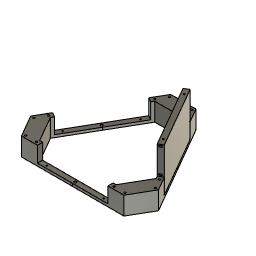
mpminideltaBase v6 (Autodesk Fusion 360 design; units mm, degrees)
Autodesk Fusion 360 part; units mm, degrees
sketch "Sketch1" plane through (0, 0, 0) normal (0, 0, 1) x (1, 0, 0)
  line L0 (0, 128.5246) -> (24.5, 128.5246)
  line L1 (24.5, 128.5246) -> (33.9962, 112.0679)
  line L2 (33.9962, 112.0679) -> (22.7364, 105.5705)
  line L3 (22.7364, 105.5705) -> (0, 105.5705)
  circle A0 centre (0, 0) radius 15
  line L4 (24.5, 128.5246) -> (25.9994, 125.9262)
  line L5 (24.5, 128.5246) -> (21.5, 128.5246)
  line L6 (33.9962, 112.0679) -> (29.6655, 109.5689)
  line L7 (33.9962, 112.0679) -> (36.4952, 107.7372)
  circle A1 centre (21.5, 123.3299) radius 1.75
  circle A2 centre (32.1825, 105.2486) radius 1.75
  line L8 (36.4952, 107.7372) -> (44.2521, 94.2946)
  line L9 (36.4952, 107.7372) -> (45.6165, 91.9302)
  line L10 (47.3658, 88.8987) -> (43.0351, 86.3997)
  line L11 (41.2858, 89.4312) -> (45.6165, 91.9302)
  arc A3 (41.2858, 89.4312) -> (43.0351, 86.3997) centre (42.1605, 87.9154) ccw
  line L12 (36.4952, 107.7372) -> (45.6165, 91.9302)
  line L13 (47.3658, 88.8987) -> (48.5676, 86.8161)
  line L14 (24.5, 128.5246) -> (45.6165, 91.9302)
  line L15 (47.3658, 88.8987) -> (74, 42.7422)
  line L16 (36.4952, 107.7372) -> (45.6165, 91.9302)
  line L17 (47.3658, 88.8987) -> (48.5676, 86.8161)
  line L18 (21.5, 123.3299) -> (21.4713, 123.3133)
  line L19 (-47.3658, 88.8987) -> (-74, 42.7422)
  line L20 (-47.3658, 88.8987) -> (-43.0351, 86.3997)
  arc A4 (-43.0351, 86.3997) -> (-41.2858, 89.4312) centre (-42.1605, 87.9154) ccw
  line L21 (-41.2858, 89.4312) -> (-45.6165, 91.9302)
  line L22 (-36.4952, 107.7372) -> (-45.6165, 91.9302)
  line L23 (-24.5, 128.5246) -> (-45.6165, 91.9302)
  circle A5 centre (-32.1825, 105.2486) radius 1.75
  line L24 (-33.9962, 112.0679) -> (-22.7364, 105.5705)
  line L25 (-22.7364, 105.5705) -> (0, 105.5705)
  circle A6 centre (-21.5, 123.3299) radius 1.75
  line L26 (0, 128.5246) -> (-24.5, 128.5246)
  line L27 (-53.3056, -85.4693) -> (-0.0159, -85.457)
  arc A7 (-53.3067, -80.4693) -> (-56.8067, -80.4701) centre (-55.0567, -80.4697) ccw
  line L28 (-56.8067, -80.4701) -> (-56.8056, -85.4701)
  line L29 (-53.3056, -85.4693) -> (-53.3067, -80.4693)
  line L30 (-98.0926, -8.961) -> (-102.4221, -6.46)
  line L31 (-100.6714, -3.4293) -> (-99.4687, -1.3473)
  arc A8 (-98.0926, -8.961) -> (-96.3419, -5.9303) centre (-97.2172, -7.4457) ccw
  line L32 (-100.6714, -3.4293) -> (-96.3419, -5.9303)
  line L33 (-100.6714, -3.4293) -> (-99.4687, -1.3473)
  line L34 (-100.6714, -3.4293) -> (-74.0159, 42.7148)
  line L35 (-111.5508, -22.2629) -> (-103.7876, -8.8238)
  circle A9 centre (-107.2392, -24.7535) radius 1.75
  line L36 (-114.0518, -26.5924) -> (-111.5508, -22.2629)
  line L37 (-123.5556, -43.0447) -> (-114.0518, -26.5924)
  circle A10 centre (-117.5568, -43.0454) radius 1.75
  line L38 (-111.3056, -64.2623) -> (-123.5556, -43.0447)
  line L39 (-111.3056, -64.2623) -> (-99.0556, -85.4799)
  line L40 (-99.0556, -85.4799) -> (-56.8056, -85.4701)
  circle A11 centre (-96.0568, -80.2845) radius 1.75
  circle A12 centre (-75.0567, -80.4951) radius 1.75
  line L41 (-80.0556, -85.4755) -> (-80.0586, -72.4755)
  line L42 (-80.0586, -72.4755) -> (-91.4268, -52.7853)
  line L43 (-102.7949, -33.095) -> (-91.4268, -52.7853)
  line L44 (-114.0518, -26.5924) -> (-102.7949, -33.095)
  line L45 (100.6714, -3.4293) -> (74.0159, 42.7148)
  arc A13 (96.3419, -5.9303) -> (98.0926, -8.961) centre (97.2172, -7.4457) ccw
  line L46 (98.0926, -8.961) -> (102.4221, -6.46)
  line L47 (100.6714, -3.4293) -> (96.3419, -5.9303)
  line L48 (56.8067, -80.4701) -> (56.8056, -85.4701)
  line L49 (53.3056, -85.4693) -> (50.9011, -85.4688)
  arc A14 (56.8067, -80.4701) -> (53.3067, -80.4693) centre (55.0567, -80.4697) ccw
  line L50 (53.3056, -85.4693) -> (53.3067, -80.4693)
  line L51 (53.3056, -85.4693) -> (50.9011, -85.4688)
  line L52 (53.3056, -85.4693) -> (0.0159, -85.457)
  line L53 (75.0556, -85.4744) -> (59.5355, -85.4708)
  circle A15 centre (75.0567, -80.4951) radius 1.75
  line L54 (80.0556, -85.4755) -> (75.0556, -85.4744)
  line L55 (99.0556, -85.4799) -> (80.0556, -85.4755)
  circle A16 centre (96.0568, -80.2845) radius 1.75
  line L56 (111.3056, -64.2623) -> (99.0556, -85.4799)
  line L57 (111.3056, -64.2623) -> (123.5556, -43.0447)
  line L58 (123.5556, -43.0447) -> (102.4221, -6.46)
  circle A17 centre (117.5568, -43.0454) radius 1.75
  circle A18 centre (107.2392, -24.7535) radius 1.75
  line L59 (114.0518, -26.5924) -> (102.7949, -33.095)
  line L60 (102.7949, -33.095) -> (91.4268, -52.7853)
  line L61 (80.0586, -72.4755) -> (91.4268, -52.7853)
  line L62 (80.0556, -85.4755) -> (80.0586, -72.4755)
  line L63 (-103.7876, -8.8238) -> (-102.4221, -6.46)
  line L64 (56.8056, -85.4701) -> (59.5355, -85.4708)
  circle A19 centre (-69.6693, 40.2432) radius 2.25
  circle A20 centre (-0.017, -80.457) radius 2.25
  circle A21 centre (69.6863, 40.2138) radius 2.25
  line L65 (-102.4221, -6.46) -> (-100.6714, -3.4293)
  line L66 (-47.3658, 88.8987) -> (-45.6165, 91.9302)
  line L67 (45.6165, 91.9302) -> (47.3658, 88.8987)
  line L68 (100.6714, -3.4293) -> (102.4221, -6.46)
  line L69 (53.3056, -85.4693) -> (56.8056, -85.4701)
  line L70 (-56.8056, -85.4701) -> (-53.3056, -85.4693)
  line L71 (-38.7044, 83.9007) -> (-65.3386, 37.7442)
  line L72 (-38.7044, 83.9007) -> (-36.9551, 86.9322)
  line L73 (-18.725, 118.5246) -> (-36.9551, 86.9322)
  line L74 (0, 118.5246) -> (-18.725, 118.5246)
  line L75 (0, 118.5246) -> (18.725, 118.5246)
  line L76 (18.725, 118.5246) -> (25.3348, 107.0699)
  line L77 (25.3348, 107.0699) -> (27.8338, 102.7392)
  line L78 (27.8338, 102.7392) -> (36.9551, 86.9322)
  line L79 (36.9551, 86.9322) -> (38.7044, 83.9007)
  line L80 (38.7044, 83.9007) -> (60.3427, 46.402)
  line L81 (60.3427, 46.402) -> (111.9829, -43.0892)
  line L82 (102.6453, -59.2623) -> (112.0078, -43.046)
  line L83 (53.3079, -75.4693) -> (10.014, -75.4593)
  line L84 (53.3079, -75.4693) -> (93.2882, -75.4693)
  line L85 (102.6453, -59.2623) -> (93.2882, -75.4693)
  line L86 (-102.6453, -59.2623) -> (-112.0078, -43.046)
  line L87 (-112.0078, -43.046) -> (-105.3927, -31.5944)
  line L88 (-102.6453, -59.2623) -> (-93.2802, -75.4832)
  line L89 (-105.3927, -31.5944) -> (-65.3386, 37.7442)
  line L90 (10.014, -75.4593) -> (-93.2802, -75.4832)
  line L91 (-12.9851, 7.5092) -> (12.9946, -7.4927)
  line L92 (-0.0084, 15) -> (-0.0106, -15)
  line L93 (12.9957, 7.4908) -> (-12.9862, -7.5073)
  circle A22 centre (-106.9755, -61.7623) radius 2.25
  circle A23 centre (106.9755, -61.7623) radius 2.25
  line L94 (0, 128.5246) -> (0, 118.5246)
  circle A24 centre (0, 123.5246) radius 2.25
  line L95 (-33.9962, 112.0679) -> (-29.6655, 109.5689)
  line L96 (0, 123.5246) -> (21.6125, 123.5246)
  line L97 (-21.6125, 123.5246) -> (-29.6655, 109.5689)
  line L98 (-5, 123.5246) -> (-21.6125, 123.5246)
  line L99 (-5, 123.5246) -> (-2.25, 123.5246)
  line L100 (-19.7609, 123.5246) -> (-13.7609, 123.5246)
  line L101 (-22.5379, 121.9209) -> (-25.5367, 116.724)
  circle A25 centre (-25.5367, 116.724) radius 2.25
  circle A26 centre (-13.7609, 123.5246) radius 2.25
  line L102 (21.6125, 123.5246) -> (41.2858, 89.4312)
  line L103 (22.5379, 121.9209) -> (25.5367, 116.724)
  circle A27 centre (25.5367, 116.724) radius 2.25
  line L104 (19.7609, 123.5246) -> (13.7609, 123.5246)
  circle A28 centre (13.7609, 123.5246) radius 2.25
  circle A29 centre (-88.3176, -80.4774) radius 2.25
  circle A30 centre (-100.095, -73.6796) radius 2.25
  circle A31 centre (-113.8559, -49.845) radius 2.25
  circle A32 centre (-113.8543, -36.2466) radius 2.25
  circle A33 centre (113.8543, -36.2466) radius 2.25
  circle A34 centre (113.8559, -49.845) radius 2.25
  circle A35 centre (100.095, -73.6796) radius 2.25
  circle A36 centre (88.3176, -80.4774) radius 2.25
  line L105 (-0.0159, -85.457) -> (0.0159, -85.457)
  line L106 (-0.0151, -75.4616) -> (-0.014, -75.4616)
  line L107 (74, 42.7422) -> (74.0159, 42.7148)
  line L108 (-74.0159, 42.7148) -> (-74, 42.7422)
  line L109 (-33.9962, 112.0679) -> (-39.9938, 101.6742)
  line L110 (-39.9938, 101.6742) -> (39.9938, 101.6742)
  line L111 (-68.0556, -85.4728) -> (-108.0494, -16.2015)
  line L112 (108.0494, -16.2015) -> (68.0556, -85.4728)
  line L113 (-39.9938, 101.6742) -> (-31.3324, 96.6762)
  line L114 (39.9938, 101.6742) -> (31.3324, 96.6762)
  line L115 (-68.0556, -85.4728) -> (-68.0579, -75.4728)
  line L116 (-108.0494, -16.2015) -> (-99.3903, -21.2035)
  line L117 (-107.2392, -24.7535) -> (-104.238, -19.558)
  line L118 (108.0494, -16.2015) -> (99.3607, -21.2152)
  line L119 (68.0556, -85.4728) -> (68.0556, -75.4693)
  dimension "d3" = 24.5
  dimension "d14" = 19
  dimension "d17" = 13
  dimension "d18" = 30
  dimension "d20" = 3
  dimension "d21" = 3
  dimension "d23" = 5
  dimension "d24" = 5
  dimension "d25" = 3.5
  dimension "d26" = 3.5
  dimension "d29" = 3.5
  dimension "d32" = 5
  dimension "d33" = 4.5
  dimension "d35" = 360
  dimension "d36" = 10
  dimension "d40" = 10
  dimension "d41" = 4.5
  dimension "d42" = 4.5
  dimension "d43" = 4.5
  dimension "d44" = 5
  dimension "d49" = 6
  dimension "d50" = 6
  dimension "d51" = 4.5
  dimension "d52" = 4.5
  dimension "d54" = 6
  dimension "d55" = 4.5
  dimension "d56" = 6
  dimension "d57" = 4.5
  dimension "d59" = 360
  dimension "d76" = 12
  dimension "d78" = 360
  dimension "d92" = 360
  dimension "d93" = 6
  constraint parallel L1 L14
  constraint perpendicular L2 L14
  constraint parallel L1 L4
  constraint parallel L0 L5
  constraint perpendicular L1 L6
  constraint perpendicular L6 L7
  constraint coincident L13.end L14
  constraint coincident L8.end L14
  constraint coincident L10.start L12
  constraint tangent L10 A3
  constraint perpendicular L10 L12
  constraint tangent L11 A3
  constraint perpendicular L9 L11
  constraint collinear L12 L13
  constraint collinear L14 L15
  constraint collinear L16 L17
  constraint perpendicular L30 L63
  constraint perpendicular L48 L64
  constraint coincident A0 L91.start
  constraint perpendicular L32 L65
  constraint perpendicular L21 L66
  constraint perpendicular L46 L68
  constraint perpendicular L50 L69
  constraint perpendicular L29 L70
  constraint parallel L80 L81
  constraint horizontal L84
  constraint collinear L82 L85
  constraint perpendicular L41 L90
  constraint collinear L86 L88
  constraint coincident L82 L81.end
  constraint coincident A0 L93.end
  constraint coincident A0 L92.start
  constraint coincident A0 L91.end
  constraint coincident L90 L106.end
  constraint coincident A0 L92.end
  constraint coincident L90 L106.start
  constraint coincident A0 L93.start
  constraint midpoint L94 A24.centre
  constraint perpendicular L73 L95
  constraint coincident A24 L99.end
  constraint parallel L98 L99
  constraint coincident A6 L100.start
  constraint coincident L98 L100.start
  constraint parallel L98 L100
  constraint coincident A6 L101.start
  constraint coincident L97 L101.start
  constraint parallel L97 L101
  constraint coincident L101.end A25.centre
  constraint coincident L100.end A26.centre
  constraint coincident A1 L103.start
  constraint coincident L102 L103.start
  constraint parallel L102 L103
  constraint coincident L103.end A27.centre
  constraint coincident A1 L104.start
  constraint coincident L96 L104.start
  constraint parallel L96 L104
  constraint coincident L104.end A28.centre
  constraint horizontal L105
  constraint perpendicular L95 L109
  constraint horizontal L110
  constraint coincident L8 L110.end
  constraint coincident L73 L113.end
  constraint perpendicular L73 L113
  constraint coincident L78 L114.end
  constraint perpendicular L78 L114
  constraint coincident A9.centre L117.start
  constraint parallel L35 L117
  constraint coincident L81 L118.end
  constraint perpendicular L81 L118
  constraint coincident L84 L119.end
  constraint perpendicular L84 L119
  measures "d3" distance of L0.start L0.end
  measures "d14" distance of L0.end L1.end
  measures "d17" distance of L1.end L2.end
  measures "d18" diameter of A0
  measures "d20" distance of L0.end L4.end
  measures "d21" distance of L0.end L5.end
  measures "d23" distance of L1.end L6.end
  measures "d24" distance of L1.end L7.end
  measures "d25" diameter of A1
  measures "d26" diameter of A2
  measures "d29" diameter of A3
  measures "d32" distance of L19.end A19.centre
  measures "d33" diameter of A19
  measures "d41" diameter of A22
  measures "d42" diameter of A23
  measures "d43" diameter of A24
  measures "d44" distance of L24.start L95.end
  measures "d49" distance of L100.start L100.end
  measures "d50" distance of L101.start L101.end
  measures "d51" diameter of A25
  measures "d52" diameter of A26
  measures "d54" distance of L103.start L103.end
  measures "d55" diameter of A27
  measures "d56" distance of L104.start L104.end
  measures "d57" diameter of A28
  measures "d76" distance of L24.start L109.end
  measures "d93" distance of A9.centre L117.end
extrude "Extrude2" add sketch "Sketch1" against normal blind 5 contours L23 L24 A6 L26 L94 A24 L95 L97 L98 L99 L100 L101 A25 A26 | L0 L1 L2 L4 L5 L6 A1 L14 L94 A24 L96 L102 L103 A27 L104 A28 | L22 L23 L24 L73 L95 L109 L110 | L2 A1 L75 L76 L94 A24 L96 L102 L103 A27 L104 A28 | L24 A6 L73 L74 L94 A24 L97 L98 L99 L100 L101 A25 A26 | L2 L6 L7 A2 L8 L9 L12 L14 L16 L102 L110 | L19 L20 A4 L21 L22 L23 L30 L31 A8 L32 L33 L34 L35 L63 L71 L72 L73 L89 L108 L113 L116 | L73 L110 L113 | L2 L3 L24 L25 L73 L74 L75 L76 | L2 A2 L77 L78 L102 L110 | L20 A4 L21 L66 | L102 L110 L114 | L8 L9 L11 L12 L14 L16 L102 L114 | L78 L102 L110 L114 | L10 A3 L13 L15 L17 L45 A13 L46 L47 L58 L78 L79 L80 L81 L102 L107 L114 L118 | L10 L11 A3 L67 | L89 L111 L116 | L30 A8 L32 L65 | L35 L36 L44 L89 L111 | L81 L112 L118 | L37 L38 L39 L40 L41 L44 L86 L87 L88 L90 | L41 L42 L43 L44 L86 L87 L88 L90 | L40 L41 L90 L111 | L90 L111 L115 | L58 L59 L81 L112 | L59 L60 L61 L62 L81 L84 L112 | L27 A7 L28 L29 L40 L48 L49 A14 L50 L51 L52 L53 L64 L83 L84 L90 L105 L115 L119 | A13 L46 L47 L68 | L59 L60 L61 L62 L81 L82 L84 L85 | L55 L56 L57 L58 L59 L62 L81 L82 L84 L85 | L84 L112 L119 | L53 L54 L62 L84 L112 | A7 L28 L29 L70 | L48 A14 L50 L69 | A10 | A11 | A16 | A17 | A22 | A23 | A29 | A30 | A31 | A32 | A33 | A34 | A35 | A36 makes body 1
extrude "Extrude3" add sketch "Sketch1" along normal blind 30 separate body contours L23 L24 A6 L26 L94 A24 L95 L97 L98 L99 L100 L101 A25 A26 | L0 L1 L2 L4 L5 L6 A1 L14 L94 A24 L96 L102 L103 A27 L104 A28 | L2 A1 L75 L76 L94 A24 L96 L102 L103 A27 L104 A28 | L24 A6 L73 L74 L94 A24 L97 L98 L99 L100 L101 A25 A26 | L2 L3 L24 L25 L73 L74 L75 L76 | L37 L38 L39 L40 L41 L44 L86 L87 L88 L90 | L41 L42 L43 L44 L86 L87 L88 L90 | L59 L60 L61 L62 L81 L82 L84 L85 | L55 L56 L57 L58 L59 L62 L81 L82 L84 L85 makes body 2 at (-107.2223, -71.3348, 10) makes body 3 at (-8.1667, 128.5246, 20) makes body 4 at (115.3889, -57.1898, 20)
extrude "Extrude4" add sketch "Sketch1" along normal blind 30 contours L94 A24 L96 | L94 A24 | L94 A24 L96 | L96 L104 A28 | L96 L104 A28 | L97 L101 A25 | L97 L101 A25 | L98 L100 A26 | L98 L100 A26 | L102 L103 A27 | L102 L103 A27 | A22 | A23 | A29 | A30 | A31 | A32 | A33 | A34 | A35 | A36 bodies 1 2 3 4
sketch "Sketch2" plane through (0, 0, 0) normal (0, 0, 1) x (1, 0, 0)
  circle A0 centre (-42.1605, 87.9154) radius 1.25
  circle A1 centre (-97.2172, -7.4457) radius 1.25
  circle A2 centre (-55.0567, -80.4697) radius 1.25
  circle A3 centre (55.0567, -80.4697) radius 1.25
  circle A4 centre (97.2172, -7.4457) radius 1.25
  circle A5 centre (42.1605, 87.9154) radius 1.25
  point P0 (-42.1605, 87.9154)
  point P1 (-97.2172, -7.4457)
  point P2 (-55.0567, -80.4697)
  point P3 (55.0567, -80.4697)
  point P4 (97.2172, -7.4457)
  point P5 (42.1605, 87.9154)
  dimension "d68" = 2.5
  dimension "d69" = 2.5
  dimension "d70" = 2.5
  dimension "d71" = 2.5
  dimension "d72" = 2.5
  dimension "d73" = 2.5
  constraint coincident P0 A0.centre
  constraint coincident P1 A1.centre
  constraint coincident P2 A2.centre
  constraint coincident P3 A3.centre
  constraint coincident P4 A4.centre
  constraint coincident P5 A5.centre
  measures "d68" diameter of A0
  measures "d69" diameter of A1
  measures "d70" diameter of A2
  measures "d71" diameter of A3
  measures "d72" diameter of A4
  measures "d73" diameter of A5
extrude "Extrude5" cut sketch "Sketch2" against normal blind 5 bodies 1
extrude "Extrude6" add sketch "Sketch1" along normal blind 30 contours L22 L23 L24 L73 L95 L109 L110 | L2 L6 L7 A2 L8 L9 L12 L14 L16 L102 L110 | L2 A2 L77 L78 L102 L110 | L35 L36 L44 L89 L111 | L40 L41 L90 L111 | L58 L59 L81 L112 | L53 L54 L62 L84 L112 bodies 1
sketch "Sketch3" plane through (0, 0, -5) normal (0, 0, -1) x (1, 0, 0)
  circle A0 centre (97.2172, 7.4457) radius 1.25
  circle A1 centre (-97.2172, 7.4457) radius 1.25
  circle A2 centre (55.0567, 80.4697) radius 1.25
  circle A3 centre (42.1605, -87.9154) radius 1.25
  circle A4 centre (-42.1605, -87.9154) radius 1.25
  circle A5 centre (-55.0567, 80.4697) radius 1.25
  line L0 (-74, -42.7422) -> (-24.5, -128.5246)
  line L1 (-24.5, -128.5246) -> (24.5, -128.5246)
  line L2 (24.5, -128.5246) -> (74, -42.7422)
  line L3 (74, -42.7422) -> (74.0159, -42.7148)
  line L4 (74.0159, -42.7148) -> (123.5556, 43.0447)
  line L5 (123.5556, 43.0447) -> (99.0556, 85.4799)
  line L6 (99.0556, 85.4799) -> (0.0159, 85.457)
  line L7 (0.0159, 85.457) -> (-0.0159, 85.457)
  line L8 (-0.0159, 85.457) -> (-99.0556, 85.4799)
  line L9 (-99.0556, 85.4799) -> (-123.5556, 43.0447)
  line L10 (-123.5556, 43.0447) -> (-74.0159, -42.7148)
  line L11 (-74.0159, -42.7148) -> (-74, -42.7422)
  line L12 (-65.3386, -37.7442) -> (-105.3927, 31.5944)
  line L13 (-105.3927, 31.5944) -> (-102.7949, 33.095)
  line L14 (-102.7949, 33.095) -> (-80.0586, 72.4755)
  line L15 (-80.0586, 72.4755) -> (-80.0579, 75.4802)
  line L16 (-80.0579, 75.4802) -> (10.014, 75.4593)
  line L17 (10.014, 75.4593) -> (53.3079, 75.4693)
  line L18 (53.3079, 75.4693) -> (73.8311, 75.4693)
  line L19 (73.8311, 75.4693) -> (102.2569, 26.2343)
  line L20 (102.2569, 26.2343) -> (25.3348, -107.0699)
  line L21 (25.3348, -107.0699) -> (22.7364, -105.5705)
  line L22 (22.7364, -105.5705) -> (-22.7364, -105.5705)
  line L23 (-22.7364, -105.5705) -> (-25.3348, -107.0699)
  line L24 (-25.3348, -107.0699) -> (-65.3386, -37.7442)
  circle A6 centre (-75.0567, 80.4951) radius 1.75
  circle A7 centre (75.0567, 80.4951) radius 1.75
  circle A8 centre (-0.017, 80.457) radius 2.25
  circle A9 centre (-13.7609, -123.5246) radius 2.25
  circle A10 centre (-69.6693, -40.2432) radius 2.25
  circle A11 centre (-107.2392, 24.7535) radius 1.75
  circle A12 centre (-32.1825, -105.2486) radius 1.75
  circle A13 centre (0, -123.5246) radius 2.25
  circle A14 centre (25.5367, -116.724) radius 2.25
  circle A15 centre (13.7609, -123.5246) radius 2.25
  circle A16 centre (107.2392, 24.7535) radius 1.75
  circle A17 centre (69.6863, -40.2138) radius 2.25
  circle A18 centre (21.5, -123.3299) radius 1.75
  circle A19 centre (-25.5367, -116.724) radius 2.25
  circle A20 centre (-21.5, -123.3299) radius 1.75
  circle A21 centre (32.1825, -105.2486) radius 1.75
  circle A22 centre (32.1825, -105.2486) radius 3
  circle A23 centre (21.5, -123.3299) radius 3
  circle A24 centre (-21.5, -123.3299) radius 3
  circle A25 centre (-32.1825, -105.2486) radius 3
  circle A26 centre (0, 0) radius 15
  circle A27 centre (107.2392, 24.7535) radius 3
  circle A28 centre (117.5568, 43.0454) radius 3
  circle A29 centre (96.0568, 80.2845) radius 3
  circle A30 centre (75.0567, 80.4951) radius 3
  circle A31 centre (-75.0567, 80.4951) radius 3
  circle A32 centre (-96.0568, 80.2845) radius 3
  circle A33 centre (-117.5568, 43.0454) radius 3
  circle A34 centre (-107.2392, 24.7535) radius 3
  dimension "d81" = 6
  dimension "d82" = 6
  dimension "d83" = 6
  dimension "d84" = 6
  dimension "d103" = 360
  constraint concentric A21 A22
  constraint concentric A18 A23
  constraint concentric A20 A24
  constraint concentric A12 A25
  constraint coincident A26.centre origin
  measures "d81" diameter of A22
  measures "d82" diameter of A23
  measures "d83" diameter of A24
  measures "d84" diameter of A25
extrude "Extrude7" cut sketch "Sketch1" against normal blind 70 contours A10 | A11 | A16 | A17 bodies 1
extrude "Extrude8" add sketch "Sketch1" along normal blind 30 contours L73 L110 L113 | L102 L110 L114 | L78 L102 L110 L114 | L89 L111 L116 | L81 L112 L118 | L90 L111 L115 | L84 L112 L119 bodies 1
extrude "Extrude9" cut sketch "Sketch1" against normal blind 30 contours L59 L60 L61 L62 L81 L84 L112 bodies 1
extrude "Extrude10" add sketch "Sketch1" along normal blind 30 contours L2 L3 L24 L25 L73 L77 L78 L110 | L41 L42 L43 L44 L89 L90 L111 | L59 L60 L61 L62 L81 L84 L112 bodies 1
extrude "Extrude11" add sketch "Sketch1" against normal blind 5 contours L2 L3 L24 L25 L73 L77 L78 L110 | L41 L42 L43 L44 L89 L90 L111 | L59 L60 L61 L62 L81 L84 L112 bodies 1
extrude "Extrude12" cut sketch "Sketch3" against normal blind 26 contours A22 | A23 | A24 | A25 | A27 | A28 | A29 | A30 | A31 | A32 | A33 | A34 bodies 1
extrude "Extrude13" cut sketch "Sketch1" against normal blind 5 contours A22 | A23 | A29 | A30 | A31 | A32 | A33 | A34 | A35 | A36 bodies 1
sketch "Sketch4" plane through (-34.024, 58.9629, 0) normal (0.499799, -0.866141, 0) x (0.866141, 0.499799, 0)
  line L0 (75.457, 0) -> (85.457, 0)
  line L1 (85.457, 0) -> (85.457, 30)
  line L2 (85.457, 30) -> (75.457, 30)
  line L3 (75.457, 30) -> (75.457, 0)
  line L4 (85.457, 30) -> (76.457, 30)
  line L5 (76.457, 30) -> (75.457, 30)
  line L6 (85.457, 30) -> (85.457, 84)
  line L7 (85.457, 30) -> (85.457, 0)
  line L8 (85.457, 0) -> (76.457, 0)
  line L9 (76.457, 0) -> (75.457, 0)
  line L10 (81.457, 31) -> (78.457, 31)
  line L11 (85.457, 35.5) -> (76.457, 35.5)
  line L12 (82.457, 33) -> (82.457, 34.5)
  line L13 (82.457, 33) -> (82.457, 32)
  line L14 (76.457, 31) -> (76.457, 35.5)
  line L15 (82.457, 34.5) -> (77.457, 34.5)
  line L16 (76.457, 31) -> (76.457, 30)
  line L17 (77.457, 34.5) -> (77.457, 32)
  line L18 (81.457, 31) -> (81.457, 32)
  line L19 (78.457, 32) -> (77.457, 32)
  line L20 (81.457, 32) -> (82.457, 32)
  line L21 (78.457, 31) -> (78.457, 32)
  line L22 (75.457, 30) -> (75.457, 84)
  line L23 (75.457, 84) -> (85.457, 84)
  line L24 (75.457, 57) -> (85.457, 57)
  line L25 (85.457, 84) -> (85.457, 83)
  line L26 (85.457, 83) -> (75.457, 83)
  line L27 (81.457, 83) -> (81.457, 82)
  line L28 (81.457, 82) -> (82.457, 82)
  line L29 (82.457, 81) -> (82.457, 82)
  line L30 (82.457, 81) -> (82.457, 79.5)
  line L31 (78.457, 83) -> (78.457, 82)
  line L32 (78.457, 82) -> (77.457, 82)
  line L33 (77.457, 79.5) -> (77.457, 82)
  line L34 (82.457, 79.5) -> (77.457, 79.5)
  line L35 (75.457, 30) -> (75.457, 0)
  line L36 (78.457, 32) -> (81.457, 32)
  line L37 (78.457, 82) -> (81.457, 82)
  dimension "d108" = 9
  dimension "d109" = 54
  dimension "d110" = 9
  dimension "d117" = 9
  dimension "d120" = 1
  dimension "d123" = 54
  dimension "d124" = 1
  dimension "d125" = 10
  constraint coincident L1.end L2.start
  constraint perpendicular L1 L4
  constraint coincident L2.end L3.start
  constraint perpendicular L4 L6
  constraint coincident L0.end L1.start
  constraint horizontal L8
  constraint coincident L0.start L3.end
  constraint perpendicular L6 L11
  constraint perpendicular L11 L12
  constraint perpendicular L10 L13
  constraint perpendicular L14 L15
  constraint perpendicular L10 L17
  constraint vertical L18
  constraint perpendicular L17 L19
  constraint perpendicular L13 L20
  constraint perpendicular L19 L21
  constraint perpendicular L2 L22
  constraint midpoint L22 L24.start
  constraint midpoint L6 L24.end
  constraint perpendicular L23 L25
  constraint perpendicular L6 L26
  constraint symmetric L12.start L24 L29.start
  constraint symmetric L12.end L24 L30.end
  constraint symmetric L15.end L24 L33.start
  constraint symmetric L10.start L24 L27.start
  constraint symmetric L18.end L24 L27.end
  constraint symmetric L17.end L24 L32.end
  constraint symmetric L10.end L24 L31.start
  constraint symmetric L19.start L24 L31.end
  constraint symmetric L13.end L24 L28.end
  constraint perpendicular L18 L36
  constraint perpendicular L27 L37
  measures "d108" distance of L1.end L4.end
  measures "d109" distance of L1.end L6.end
  measures "d110" distance of L0.end L8.end
  measures "d117" distance of L11.start L11.end
  measures "d120" distance of L10.start L18.end
  measures "d123" distance of L2.end L22.end
  measures "d124" distance of L6.end L25.end
  measures "d125" distance of L25.end L26.end
extrude "Extrude1" add sketch "Sketch4" along normal blind 68.5 separate body contours L0 L1 L2 L3 L4 L5 L7 L8 L9 L35 | L2 L5 L6 L11 L14 L16 L22 L24 | L2 L4 L6 L11 L14 L16 | L6 L22 L24 L26 L27 L28 L29 L30 L31 L32 L33 L34 | L6 L22 L23 L25 L26 | L26 L27 L31 L37 | L28 L29 L30 L32 L33 L34 L37 | L10 L18 L21 L36 | L12 L13 L15 L17 L19 L20 L36 makes body 5 in component "Component"
extrude "Extrude2'" cut sketch "Sketch4" along normal blind 17 contours L28 L29 L30 L32 L33 L34 L37 | L12 L13 L15 L17 L19 L20 L36 bodies 5 in component "Component"
sketch "Sketch5" plane through (0, 0, 0) normal (0, 0, -1) x (1, 0, 0)
  line L0 (31.3324, -96.6762) -> (39.9938, -101.6742)
  line L1 (39.9938, -101.6742) -> (74.23, -42.3436)
  line L2 (74.23, -42.3436) -> (65.5686, -37.3456)
  line L3 (65.5686, -37.3456) -> (31.3324, -96.6762)
  line L4 (39.9938, -101.6742) -> (31.3324, -96.6762)
  line L5 (35.6631, -99.1752) -> (42.1605, -87.9154)
  circle A0 centre (42.1605, -87.9154) radius 1.5
  circle A1 centre (42.1605, -87.9154) radius 3
  dimension "d130" = 13
  dimension "d131" = 3
  dimension "d132" = 6
  constraint coincident L0.end L1.start
  constraint coincident L0.start L3.end
  constraint midpoint L4 L5.start
  constraint perpendicular L4 L5
  constraint coincident L5.end A0.centre
  measures "d130" distance of L5.start L5.end
  measures "d131" diameter of A0
  measures "d132" diameter of A1
extrude "Extrude3'" cut sketch "Sketch5" against normal blind 32 contours A0 bodies 5 in component "Component"
extrude "Extrude4'" cut sketch "Sketch5" against normal blind 28 contours A1 bodies 5 in component "Component"
sketch "Sketch6" plane through (0, 0, 84) normal (0, 0, 1) x (-1, 0, 0)
  line L0 (-39.9938, -101.6742) -> (-31.3324, -96.6762)
  line L1 (-31.3324, -96.6762) -> (-65.5686, -37.3456)
  line L2 (-65.5686, -37.3456) -> (-74.23, -42.3436)
  line L3 (-74.23, -42.3436) -> (-39.9938, -101.6742)
  line L4 (-35.6631, -99.1752) -> (-42.1605, -87.9154)
  circle A0 centre (-42.1605, -87.9154) radius 1.5
  dimension "d137" = 13
  dimension "d138" = 3
  constraint midpoint L0 L4.start
  constraint perpendicular L0 L4
  constraint coincident L4.end A0.centre
  measures "d137" distance of L4.start L4.end
  measures "d138" diameter of A0
extrude "Extrude5'" cut sketch "Sketch6" against normal blind 2 contours A0 bodies 5 in component "Component"
sketch "Sketch7" plane through (74.0178, 42.7114, 0) normal (0.866141, 0.499799, 0) x (-0.499799, 0.866141, 0)
  line L0 (68.0754, 0) -> (68.0754, 84)
  line L1 (68.0754, 84) -> (-0.4246, 84)
  line L2 (-0.4246, 84) -> (-0.4246, 0)
  line L3 (-0.4246, 0) -> (68.0754, 0)
  line L4 (-0.4246, 84) -> (-0.3246, 84)
  line L5 (-0.3246, 84) -> (-0.3246, 82.9)
  dimension "d141" = 0.1
  constraint coincident L1.end L2.start
  constraint horizontal L4
  constraint perpendicular L4 L5
  measures "d141" distance of L1.end L4.end
ref_plane "WorkPlane1" through (69.6794, 40.2257, 42) normal (0.499799, -0.866141, 0) x (0, 0, -1)
split "Split1" by plane through (69.6794, 40.2257, 42) normal (0.499799, -0.866141, 0) bodies 5 makes body 6 at (68.4558, 39.0116, 56) in component "Component"
delete_body "RemoveBody1" bodies 6 in component "Component"
mirror "Mirror1" about plane through (69.6794, 40.2257, 42) normal (0.499799, -0.866141, 0) of bodies 5 merged in component "Component"
sketch "Sketch8" plane through (0, 0, 0) normal (0, 0, -1) x (1, 0, 0)
  circle A0 centre (97.1984, 7.4641) radius 3
  line L0 (99.3651, 21.2229) -> (31.3324, -96.6762)
  line L1 (31.3324, -96.6762) -> (39.9938, -101.6742)
  line L2 (39.9938, -101.6742) -> (108.0265, 16.2249)
  line L3 (108.0265, 16.2249) -> (99.3651, 21.2229)
  circle A1 centre (42.1605, -87.9154) radius 3
  line L4 (35.6631, -99.1752) -> (103.6958, 18.7239)
  circle A2 centre (69.6794, -40.2257) radius 2.25
  circle A3 centre (69.6794, -40.2257) radius 3
  dimension "d145" = 4.5
  dimension "d148" = 6
  constraint midpoint L1 L4.start
  constraint midpoint L3 L4.end
  constraint midpoint L4 A2.centre
  constraint concentric A2 A3
  measures "d145" diameter of A2
  measures "d148" diameter of A3
extrude "Extrude6'" cut sketch "Sketch8" against normal blind 5 contours L4 A2 | L4 A2 bodies 5 in component "Component"
extrude "Extrude7'" cut sketch "Sketch8" against normal blind 6 contours L4 A2 A3 | L4 A2 A3 | L4 A2 | L4 A2 bodies 5 in component "Component"
component "Component" placed x (1, 0, 0) y (0, 1, 0) z (0, 0, 1) at (0, 0, 0)
named bodies: "MiddleFraming"
